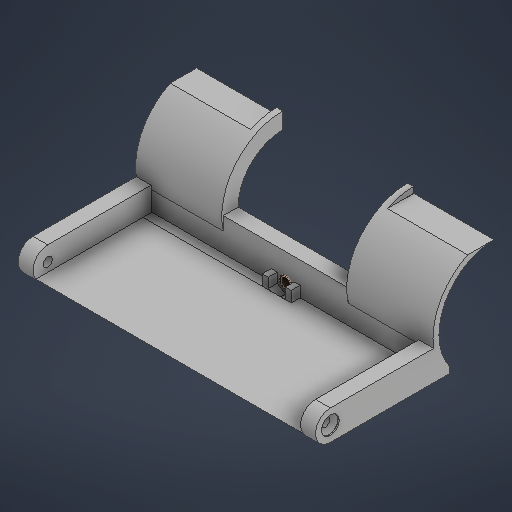
# Autodesk Inventor part: main body wheels part
Saved by Autodesk Inventor 2027 (Build 310192000, 192)
## iProperties
Created: 2026-04-17
Part Number: main body wheels part
Material: Generic
Document SubType Name: Modeling
Designer: Martin
Density: 1 g/cm^3
Appearance: Bronze - Satin
Author: Martin
Autodesk Inventor part; units mm, degrees
ref_plane "YZ Plane" through (0, 0, 0) normal (1, 0, 0) x (0, 1, 0)
ref_plane "XZ Plane" through (0, 0, 0) normal (0, 1, 0) x (-1, 0, 0)
ref_plane "XY Plane" through (0, 0, 0) normal (0, 0, 1) x (1, 0, 0)
sketch "Sketch1" plane through (0, 0, 0) normal (1, 0, 0) x (0, 1, 0)
  circle A0 centre (0, 0) radius 15
  line L0 (-13, -15) -> (-13, 85)
  arc A1 (18.5, 0) -> (-10.8282, 15) centre (0, 0) ccw
  arc A2 (18.5, 8.8318) -> (-13, 15.8509) centre (0, 0) ccw
  line L1 (18.5, 25) -> (18.5, -15) construction
  line L2 (0, 15) -> (-13, 15)
  line L3 (-10.5, 15) -> (-7.5, 15)
  line L4 (-7.5, 15) -> (-7.5, 24)
  line L5 (-7.5, 24) -> (-10.5, 24)
  line L6 (-10.5, 24) -> (-10.5, 15)
  line L7 (18.5, 8.8318) -> (18.5, 0)
  line L8 (-9, 24) -> (-9, 15) construction
  arc A3 (-10.8282, 15) -> (-13, 13.1624) centre (0, 0) ccw
  point P0 (0, -15)
  point P1 (-13, 7.4833)
  dimension "d0" = 30
  dimension "d1" = 2
  dimension "d3" = 100
  dimension "d4" = 37
  dimension "d5" = 41
  dimension "d7" = 3
  dimension "d8" = 9
  dimension "d9" = 2.5
  dimension "d10" = 15
  dimension "d11" = 40
  dimension "d12" = 18.5
  constraints: 18 end point, 9 point on circle, 6 point on line, 4 centre point, 3 coincident, 2 horizontal alignment, 2 midpoint, 2 parallel, 2 perpendicular, 2 tangent, 2 vertical, 1 horizontal
  measures "d0" diameter of A0
  measures "d1" distance edge to line of A0 L0
  measures "d3" distance of L0.start L0.end
  measures "d4" diameter of A1
  measures "d5" diameter of A2
  measures "d7" distance of L5.end L4.end
  measures "d8" distance of L5.end L3.start
  measures "d9" distance between parallel lines of L0 L6
  measures "d10" vertical distance of point (0, 0) L0.start
  measures "d11" distance of L1.end L1.start
  measures "d12" distance of A0.start L1.end
extrude "Extrusion1" add sketch "Sketch1" along normal mid plane 100 contours A0 L0 | A0 L0
extrude "Extrusion2" add sketch "Sketch1" along normal mid plane 49 contours A0 L0 A3 L2 | L0 L2 A3
sketch "Sketch2" plane through (-24.5, -13, 15) normal (0, 0, 1) x (1, 0, 0)
  circle A0 centre (24.5, 4) radius 1.5
  point P0 (24.5, 13)
  constraints: 1 centre point
extrude "Extrusion3" add sketch "Sketch2" along normal blind 9
sketch "Sketch3" plane through (-24.5, -13, 15) normal (0, 0, 1) x (1, 0, 0)
  circle A0 centre (24.5, 4) radius 1.5 projected
  circle A1 centre (24.5, 4) radius 1.55
  circle A2 centre (24.5, 4) radius 2.05
  point P0 (24.5, 13)
  dimension "d25" = 3.1
  dimension "d26" = 4.1
  constraints: 4 coincident, 2 centre point
  measures "d25" diameter of A1
  measures "d26" diameter of A2
extrude "Extrusion4" add sketch "Sketch3" along normal blind 5 separate body contours A2
extrude "Extrusion5" cut sketch "Sketch1" along normal mid plane 50 contours A0 L0 | A0 L0 bodies 1
extrude "Extrusion6" add sketch "Sketch1" against normal blind 27 from surface at 50 separate body contours L4 A2 L7 A1 | A1 L6 A2 L4 | L0 A2 L6 A1 L2
extrude "Extrusion7" add sketch "Sketch1" along normal blind 27 from surface at -50 contours L4 A2 L7 A1 | A1 L6 A2 L4 | L0 A2 L6 A1 L2 bodies 3
sketch "Sketch4" plane through (-24.5, -13, 15) normal (0, 0, 1) x (1, 0, 0)
  circle A0 centre (24.5, 4) radius 2.075
  line L0 (1.5, 2.1718) -> (1.5, 0) projected
  line L1 (47.5, 31.5) -> (47.5, 0) projected
  line L2 (1.5, 0) -> (47.5, 0)
  line L3 (47.5, 0) -> (47.5, 13)
  line L4 (47.5, 13) -> (1.5, 13)
  line L5 (1.5, 13) -> (1.5, 0)
  point P0 (24.5, 13)
  point P1 (47.5, 0)
  dimension "d30" = 4.15
  constraints: 8 end point, 2 parallel, 1 centre point, 1 horizontal, 1 perpendicular, 1 point on line
  measures "d30" diameter of A0
sketch "Sketch5" plane through (50, -13, 15) normal (1, 0, 0) x (0, 0, -1)
  arc A0 (6.1682, 31.5) -> (-0.8509, 0) centre (15, 13) ccw projected
  arc A1 (15, 31.5) -> (0, 2.1718) centre (15, 13) ccw projected
  line L0 (0, 0) -> (-0.8509, 0) projected
  line L1 (0, 0) -> (7.5167, 0) projected
  line L2 (0, 2.1718) -> (0, 0) projected
  line L3 (0, 31.5) -> (0, 0) projected
  line L4 (0, 13) -> (0, 0) projected
extrude "Extrusion8" add sketch "Sketch4" along normal blind 5 bodies 3
sketch "Sketch6" plane through (23, -13, 20) normal (1, 0, 0) x (0, 0, -1)
  arc A0 (11.1682, 31.5) -> (4.1491, 0) centre (20, 13) ccw projected
  line L0 (4.1491, 0) -> (0, 0) projected
  line L1 (0, 0) -> (0, 8.5)
  line L2 (0, 13) -> (0, 8.5) projected
  line L3 (0, 0) -> (4.1491, 0)
  constraints: 4 end point, 1 collinear, 1 perpendicular, 1 point on circle
extrude "Extrusion9" add sketch "Sketch6" along normal blind 27 bodies 3
extrude "Extrusion10" add sketch "Sketch6" against normal blind 27 from surface at -46 bodies 3
sketch "Sketch7" plane through (23, 18.5, 0) normal (-1, 0, 0) x (0, 0, 1)
  arc A0 (18.5, -18.5) -> (0, 0) centre (0, -18.5) ccw projected
  line L0 (8.8318, 0) -> (0, 0) projected
  arc A1 (15.8509, -31.5) -> (8.8318, 0) centre (0, -18.5) ccw projected
  line L1 (0, 0) -> (-21, 0)
  circle A2 centre (0, -18.5) radius 18.5
  constraints: 2 end point, 1 centre point, 1 coincident, 1 concentric, 1 point on line, 1 tangent
sketch "Sketch8" plane through (-24.5, -13, 20) normal (0, 0, 1) x (1, 0, 0)
  line L0 (21.75, 5.5875) -> (21.75, 2.4125)
  line L1 (21.75, 2.4125) -> (21.75, 5.5875)
  circle A0 centre (24.5, 4) radius 2.075 projected
  line L2 (-25.5, 8.5) -> (1.5, 8.5) projected
  line L3 (-25.5, 8.5) -> (-25.5, 0) projected
  line L4 (74.5, 0) -> (-25.5, 0) projected
  line L5 (74.5, 8.5) -> (74.5, 0) projected
  line L6 (47.5, 8.5) -> (74.5, 8.5) projected
  line L7 (47.5, 13) -> (47.5, 8.5) projected
  line L8 (47.5, 13) -> (1.5, 13) projected
  line L9 (1.5, 8.5) -> (1.5, 13) projected
  circle A1 centre (24.5, 4) radius 2.05 projected
  circle A2 centre (24.5, 4) radius 1.55 projected
  circle A3 centre (24.5, 4) radius 1.5 projected
  line L10 (21.7502, 2.4122) -> (24.4998, 0.8247)
  line L11 (24.5002, 0.8247) -> (27.2498, 2.4122)
  line L12 (27.25, 2.4125) -> (27.25, 5.5875)
  line L13 (27.2498, 5.5878) -> (24.5002, 7.1753)
  line L14 (24.4998, 7.1753) -> (21.7502, 5.5878)
  line L15 (74.5, 0) -> (-25.5, 0)
  line L16 (-25.5, 0) -> (-25.5, 2)
  line L17 (74.5, 1.9999) -> (74.5, 0)
  line L18 (27.2498, 5.5878) -> (21.7502, 2.4122) construction
  line L19 (27.2498, 5.5878) -> (27.25, 5.5879)
  line L20 (24.5, 4) -> (27.25, 2.4125) construction
  line L21 (27.25, 2.4125) -> (27.2502, 2.4124)
  line L22 (27.35, 5.6454) -> (27.35, 2.3546)
  line L23 (24.5, 7.2909) -> (27.35, 5.6454)
  line L24 (21.65, 5.6454) -> (24.5, 7.2909)
  line L25 (21.65, 2.3546) -> (21.65, 5.6454)
  line L26 (24.5, 0.7091) -> (21.65, 2.3546)
  line L27 (27.35, 2.3546) -> (24.5, 0.7091)
  line L28 (29.3502, 1.9999) -> (74.5, 1.9999)
  line L29 (-25.5, 2) -> (22.2641, 2)
  line L30 (29.3502, 1.9999) -> (29.3502, 5.6454)
  line L31 (29.3502, 5.6454) -> (27.35, 5.6454)
  line L32 (19.65, 2) -> (19.65, 5.6454)
  line L33 (19.65, 5.6454) -> (21.65, 5.6454)
  line L34 (29.3502, 1.9999) -> (26.7357, 1.9999)
  line L35 (27.35, 5.6454) -> (27.35, 2.3546)
  line L36 (27.3498, 2.3544) -> (26.7357, 1.9999)
  line L37 (21.65, 5.6454) -> (21.65, 2.3546)
  line L38 (21.65, 2.3546) -> (22.2641, 2)
  point P0 (24.5, 13)
  point P1 (27.35, 2.3546)
  point P2 (21.65, 2.3546)
  point P3 (24.5, 0.7091)
  point P4 (74.5, 1.9999)
  dimension "d45" = 360
  dimension "d47" = 1.5875
  dimension "d48" = 1.5875
  dimension "d49" = 2.75
  dimension "d50" = 2
  dimension "d51" = 0.1
  dimension "d54" = 360
  dimension "d56" = 2.0002
  dimension "d57" = 3.6456
  dimension "d59" = 2
  constraints: 62 end point, 7 point on line, 6 parallel, 5 perpendicular, 2 horizontal, 2 vertical, 1 collinear, 38 other
  measures "d47" vertical distance of A1.centre L0.start
  measures "d48" vertical distance of L0.end point (24.5, 4)
  measures "d49" distance from line of A0.centre L0
  measures "d50" distance of L15.end L16.end
  measures "d51" distance between parallel lines of L12 L22
  measures "d56" distance of L30.end L23.end
  measures "d57" distance of L28.start L30.end
  measures "d59" distance of L32.end L25.end
extrude "Extrusion11" add sketch "Sketch8" along normal blind 3 contours L32 L33 L25 L26 L29 | L34 L27 L22 L31 L30 bodies 3
extrude "Extrusion12" add sketch "Sketch8" along normal blind 3 contours L29 L26 L27 L34 L28 L5 L4 L3 bodies 3
sketch "Sketch9" plane through (50, -13, 15) normal (1, 0, 0) x (0, 0, -1)
  line L0 (6.1682, 31.5) -> (15, 31.5) projected
  line L1 (6.1682, 31.5) -> (-11, 31.5)
  arc A0 (6.1682, 31.5) -> (-5, 8.5) centre (15, 13) ccw projected
  line L2 (-5.5, 13) -> (-5.5, 31.5)
  arc A1 (6.1682, 31.5) -> (-5, 8.5) centre (15, 13) ccw projected
  arc A2 (15, 31.5) -> (0, 2.1718) centre (15, 13) ccw projected
  line L3 (0, 31.5) -> (0, 26.9732)
  constraints: 6 end point, 2 point on circle, 2 point on line, 1 horizontal, 1 perpendicular, 1 tangent, 1 vertical
sketch "Sketch10" plane through (50, -13, 15) normal (1, 0, 0) x (0, 0, -1)
  arc A0 (15, 31.5) -> (0, 2.1718) centre (15, 13) ccw projected
  arc A1 (0, 2.1718) -> (1.8376, 0) centre (15, 13) ccw projected
  line L0 (0, 0) -> (-8, 0) projected
  line L1 (0, 0) -> (-40, 0)
  arc A2 (-40, 10) -> (-40, 0) centre (-40, 5) ccw
  line L2 (-40, 10) -> (-5, 10)
  line L3 (-5, 6.05) -> (-5, 1.95) projected
  line L4 (-5, 10) -> (-5, 1.95)
  line L5 (-8, 0) -> (-8, 1.9999) projected
  line L6 (-5, 1.95) -> (-8, 1.9999)
  line L7 (-8, 1.9999) -> (-8, 0)
  line L8 (-8, 1.9999) -> (-8, 5.6454) projected
  point P0 (-5, 6.05)
  point P1 (-45, 5)
  dimension "d85" = 10
  dimension "d86" = 37
  constraints: 10 end point, 3 point on circle, 2 collinear, 2 horizontal, 2 tangent, 1 centre point
  measures "d85" distance between parallel lines of L1 L2
  measures "d86" distance from line of L8 point (-45, 5)
extrude "Extrusion13" add sketch "Sketch10" against normal blind 5 bodies 3
extrude "Extrusion14" add sketch "Sketch10" along normal blind 5 from surface at -100 bodies 3
sketch "Sketch11" plane through (-24.5, -13, 23) normal (0, 0, 1) x (1, 0, 0)
  line L0 (-20.5, 0) -> (69.5, 0) projected
  line L1 (69.5, 0) -> (69.5, 1.9999) projected
  line L2 (-20.5, 0) -> (69.5, 0)
  line L3 (69.5, 0) -> (69.5, 1.9999)
  line L4 (69.5, 1.9999) -> (-20.5, 1.9999)
  line L5 (-20.5, 1.9999) -> (-20.5, 0)
  point P0 (24.5, 13)
  constraints: 8 end point, 2 parallel, 1 horizontal, 1 perpendicular
extrude "Extrusion15" add sketch "Sketch11" along normal blind 62 bodies 3
sketch "Náčrt12" plane through (50, -13, 15) normal (1, 0, 0) x (0, 0, -1)
  arc A0 (-40, 10) -> (-40, 0) centre (-40, 5) ccw projected
  line L0 (0, 0) -> (-40, 0) projected
  line L1 (-40, 0) -> (-70, 0)
  arc A1 (-43.9999, 1.9999) -> (-40, 0) centre (-40, 5) ccw projected
  line L2 (-70, 0) -> (-70, 10)
  line L3 (-70, 10) -> (-40, 10)
  point P0 (15, 13)
  constraints: 6 end point, 3 tangent, 2 perpendicular, 1 horizontal
extrude "Vysunutí16" cut sketch "Náčrt12" against normal through all bodies 3
sketch "Náčrt13" plane through (-23, 18.5, 8.8318) normal (1, 0, 0) x (0, 0, -1)
  arc A0 (0, 0) -> (-11.1682, -23) centre (8.8318, -18.5) ccw projected
  line L0 (-6.1682, -18.5) -> (-6.1682, -29.3282) projected
  circle A1 centre (8.8318, -18.5) radius 15
  line L1 (-6.1682, -18.5) -> (-9.6682, -18.5) projected
  line L2 (-6.1682, -18.5) -> (-11.1682, -18.5)
  line L3 (-11.1682, -18.5) -> (-11.1682, -23)
  line L4 (8.8318, 0) -> (8.8318, -3.5)
  line L5 (8.8318, 0) -> (8.8318, 2)
  arc A2 (8.8318, 2) -> (0, 0) centre (8.8318, -18.5) ccw
  line L6 (-11.1682, -18.5) -> (-9.6682, -18.5) projected
  point P0 (8.8318, 1)
  dimension "d73" = 2
  dimension "d74" = 3.5
  constraints: 8 end point, 6 point on circle, 2 centre point, 2 perpendicular, 2 vertical, 1 coincident, 1 collinear, 1 concentric, 1 midpoint, 1 vertical alignment
  measures "d73" distance of L4.start L5.end
  measures "d74" distance of L4.start L4.end
extrude "Vysunutí17" add sketch "Náčrt13" along normal blind 2 contours A2 L5 L4 A1 L1 L2 L3 A0 bodies 3
extrude "Vysunutí18" add sketch "Náčrt13" against normal blind 2 from surface at 46 contours A2 L5 L4 A1 L1 L2 L3 A0 bodies 3
sketch "Náčrt17" plane through (50, -13, 15) normal (1, 0, 0) x (0, 0, -1)
  circle A0 centre (-40, 5) radius 3
  point P0 (15, 13)
  dimension "d101" = 6
  constraints: 1 centre point
  measures "d101" diameter of A0
extrude "Vysunutí21" cut sketch "Náčrt17" against normal blind 0.4 bodies 3
extrude "Vysunutí22" cut sketch "Náčrt17" along normal blind 0.4 from surface at -100 bodies 3
sketch "Náčrt18" plane through (49.6, -8, 55) normal (1, 0, 0) x (0, 0, -1)
  circle A0 centre (0, 0) radius 3 projected
  point P0 (55, 8)
  point P1 (3, 0)
  constraints: 2 horizontal alignment, 1 other
hole "Díra4" at (49.6, -8, 55) direction (-1, 0, 0) diameter 3.1 depth 4.6 countersink diameter 5.8 countersink angle 90 bodies 3
sketch "Náčrt19" plane through (-49.6, -8, 55) normal (-1, 0, 0) x (0, 0, 1)
  point P0 (-55, 8)
  point P1 (0, 0)
hole "Díra5" at (-49.6, -8, 55) direction (1, 0, 0) diameter 3.1 depth 4.6 countersink diameter 5.8 countersink angle 90 bodies 3
equation "\"d48\" = d47"
body "Solid3"
